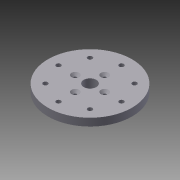
# Autodesk Inventor part: ToolHolderAdapter
Saved by Autodesk Inventor 2012 SP1 (Build 160190100, 190)
## iProperties
Created: 2010-03-22
Part Number: ToolHolderAdapter
Document SubType Name: Modeling
Designer: rconnaug
Density: 2.71 g/cm^3
Material: Aluminum-6061
Mass: 195.392 g
Surface Area: 208.903 cm^2
Volume: 72.1005 cm^3
Author: rconnaug
Autodesk Inventor part; units mm, degrees
ref_plane "YZ Plane" through (0, 0, 0) normal (1, 0, 0) x (0, 1, 0)
ref_plane "XZ Plane" through (0, 0, 0) normal (0, 1, 0) x (-1, 0, 0)
ref_plane "XY Plane" through (0, 0, 0) normal (0, 0, 1) x (1, 0, 0)
sketch "Sketch1" plane through (0, 0, 0) normal (0, 0, 1) x (1, 0, 0)
  line L0 (-10, 0) -> (60, 0) projected
  line L1 (22.5, 4.4) -> (50, 4.4)
  line L2 (50, 4.4) -> (50, 13.45)
  line L3 (50, 13.45) -> (7.5057, 13.45)
  line L4 (0, 13.45) -> (0, 0)
  line L5 (22.5, 0) -> (22.5, 4.4)
  line L6 (7.5057, 13.45) -> (7.5057, 0)
  line L7 (12.1, 0) -> (12.1, 1.2)
  line L8 (12.1, 1.2) -> (13.925, 1.2)
  line L9 (13.925, 1.2) -> (13.925, 0)
  line L10 (7.5057, 0) -> (12.1, 0)
  line L11 (13.925, 0) -> (22.5, 0)
  dimension "d0" = 4.4
  dimension "d1" = 13.45
  dimension "d2" = 45
  dimension "d3" = 100
  dimension "d28" = 15.0114
  dimension "d40" = 27.85
  dimension "d41" = 24.2
  dimension "d42" = 1.2
  constraints: 22 end point, 6 parallel, 5 perpendicular, 1 collinear, 1 point on line, 1 vertical
  measures "d0" distance between parallel lines of L0 L1
  measures "d1" distance between parallel lines of L0 L3
  measures "d2" diameter of L5 L4
  measures "d3" diameter of L2 L4
  measures "d28" diameter of L6 L4
  measures "d40" diameter of L9 L4
  measures "d41" diameter of L7 L4
  measures "d42" distance between parallel lines of L0 L8
revolve "Revolution1" add sketch "Sketch1" angle 360 about axis through (0, 13.45, 0) along (0, -1, 0) contours L6 L3 L2 L1 L5 L0 L9 L8 L7
sketch "Sketch3" plane through (0, 4.4, 0) normal (0, -1, 0) x (1, 0, 0)
  circle A0 centre (0, 0) radius 22.5 projected
  line L0 (0, -70) -> (0, 70) projected
  point P0 (0, 37.5)
  dimension "d16" = 37.5
  constraints: 1 point on line
  measures "d16" distance of A0.centre point (0, 37.5)
hole "Hole2" at (0, 4.4, 37.5) direction (0, 1, 0) diameter 5.5 end through all countersink diameter 11.4 countersink angle 90 clearance for "Flat Head Machine Screw" size "M5" standard "Ansi Metric M Profile"
pattern_circular "Circular Pattern2" count 8 over 360 about axis through (0, 8.925, 0) along (0, -1, 0) of "Hole2"
sketch "Sketch5" plane through (0, 13.45, 0) normal (0, 1, 0) x (1, 0, 0)
  circle A0 centre (0, 0) radius 50 projected
  line L0 (-70, 0) -> (70, 0) projected
  point P0 (-17.5, 0)
  dimension "d29" = 17.5
  constraints: 1 point on line
  measures "d29" distance of A0.centre point (-17.5, 0)
hole "Hole3" at (-17.5, 13.45, 0) direction (0, -1, 0) diameter 3.797 end through all countersink diameter 9 countersink angle 82 clearance for "Flat Head Machine Screw (82)" size "#6" standard "Ansi Unified Screw Threads"
pattern_circular "Circular Pattern3" count 4 over 360 about axis through (0, 8.925, 0) along (0, -1, 0) of "Hole3"
body "Solid1"
